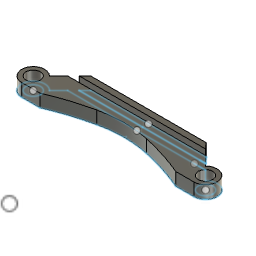
Finger1Section2P2V1 v2 (Autodesk Fusion 360 design; units mm, degrees)
Autodesk Fusion 360 part; units mm, degrees
sketch "Sketch1" plane through (0, 0, 0) normal (0, 0, 1) x (1, 0, 0)
  circle A0 centre (0.507, 0) radius 1.25
  line L0 (4.507, 4) -> (5.507, 5)
  arc A1 (1.9212, 1.4142) -> (0.507, -2) centre (0.507, 0) ccw
  line L1 (1.9212, 1.4142) -> (3.507, 3)
  line L2 (0.507, -2) -> (3.6836, -2)
  arc A2 (11.1884, 0.3961) -> (3.6836, -2) centre (20.507, -41.7412) ccw
  line L3 (26.507, 4) -> (25.5594, 4)
  line L4 (15.5594, 4) -> (4.507, 4)
  line L5 (4.507, 4) -> (15.5594, 4)
  line L6 (25.5594, 4) -> (26.507, 4)
  line L7 (5.507, 5) -> (15.5594, 5)
  line L8 (25.5594, 5) -> (25.6118, 5)
  line L9 (27.507, 3) -> (25.5594, 3)
  line L10 (15.5594, 3) -> (3.507, 3)
  arc A3 (27.3304, -2) -> (19.8257, 0.3961) centre (10.507, -41.7412) ccw
  line L11 (15.5594, 5) -> (25.6118, 5)
  circle A4 centre (30.507, 0) radius 1.25
  line L12 (27.507, 3) -> (15.5594, 3)
  line L13 (30.507, -2) -> (27.3304, -2)
  line L14 (25.6118, 5) -> (26.507, 4)
  line L15 (29.0928, 1.4142) -> (27.507, 3)
  line L16 (15.5594, 4) -> (26.507, 4)
  line L17 (26.507, 4) -> (15.5594, 4)
  line L18 (15.5594, 1.1297) -> (15.5594, 1.1174)
  arc A5 (30.507, -2) -> (29.0928, 1.4142) centre (30.507, 0) ccw
  arc A6 (19.8257, 0.3961) -> (11.1884, 0.3961) centre (15.507, -19.1321) ccw
  dimension "d3" = 2.5
  dimension "d5" = 1
  dimension "d7" = 4
  dimension "d9" = 1
  dimension "d18" = 2.5
  dimension "d19" = 4
  dimension "d20" = 20
  constraint horizontal L3
  constraint horizontal L5
  constraint horizontal L9
  constraint concentric A0 A1
  constraint parallel L3 L7
  constraint coincident L1.end L9
  constraint tangent A1 L2
  constraint coincident L8.start L7
  constraint collinear L3 L4
  constraint collinear L5 L6
  constraint collinear L7 L8
  constraint collinear L9 L10
  constraint horizontal L17
  constraint horizontal L12
  constraint tangent L13 A5
  constraint coincident L18.start A2
  constraint coincident L18.end A3
  constraint tangent A2 A6
  constraint tangent A3 A6
  measures "d3" diameter of A0
  measures "d5" distance of L5 L9
  measures "d7" diameter of A1
  measures "d9" distance of L3 L7
  measures "d18" diameter of A4
  measures "d19" diameter of A5
  measures "d20" radius of A6
extrude "Extrude3" add sketch "Sketch1" along normal blind 2.2 contours A1 L1 L2 A2 L9 L10 A3 L12 L13 L15 A5 A6 makes body 1
extrude "Extrude4" add sketch "Sketch1" along normal blind 2.2 separate body contours L0 L3 L4 L5 L6 L7 L8 L11 L14 L16 L17 makes body 2
